Autodesk Fusion 360 part; units mm, degrees
(part 5 of 5)
equation "d1224 = DeckThick"
equation "d1226 = ( FootHeight ) + PanHeight - DeckThick"
equation "d1228 = ( BaseX + LeftRun + FaucetGap + RightRun - RightSideDepth ) + ( ( RightSideDepth ) - ( ( Wall + DeckClearance + RimBorder ) + ( ( RightSideDepth ) - 2 * ( Wall + DeckClearance + RimBorder ) ) ) )"
equation "d1229 = ( BaseY + Depth + ModuleGap ) + ( ( ( ( RightReach ) - ( 14 * SlotPitch + SlotWidth ) ) / 2 ) + ( 12 * SlotPitch ) )"
equation "d1230 = ( RightSideDepth ) - 2 * ( Wall + DeckClearance + RimBorder )"
equation "d1231 = SlotWidth"
equation "d1232 = DeckThick"
equation "d1234 = ( FootHeight ) + PanHeight - DeckThick"
equation "d1236 = ( BaseX + LeftRun + FaucetGap + RightRun - RightSideDepth ) + ( ( RightSideDepth ) - ( ( Wall + DeckClearance + RimBorder ) + ( ( RightSideDepth ) - 2 * ( Wall + DeckClearance + RimBorder ) ) ) )"
equation "d1237 = ( BaseY + Depth + ModuleGap ) + ( ( ( ( RightReach ) - ( 14 * SlotPitch + SlotWidth ) ) / 2 ) + ( 13 * SlotPitch ) )"
equation "d1238 = ( RightSideDepth ) - 2 * ( Wall + DeckClearance + RimBorder )"
equation "d1239 = SlotWidth"
equation "d1240 = DeckThick"
equation "d1242 = ( FootHeight ) + PanHeight - DeckThick"
equation "d1244 = ( BaseX + LeftRun + FaucetGap + RightRun - RightSideDepth ) + ( ( RightSideDepth ) - ( ( Wall + DeckClearance + RimBorder ) + ( ( RightSideDepth ) - 2 * ( Wall + DeckClearance + RimBorder ) ) ) )"
equation "d1245 = ( BaseY + Depth + ModuleGap ) + ( ( ( ( RightReach ) - ( 14 * SlotPitch + SlotWidth ) ) / 2 ) + ( 14 * SlotPitch ) )"
equation "d1246 = ( RightSideDepth ) - 2 * ( Wall + DeckClearance + RimBorder )"
equation "d1247 = SlotWidth"
equation "d1248 = DeckThick"
equation "d1250 = TouchChamfer"
equation "d1251 = FootHeight + PanHeight - DeckThick"
equation "d1253 = ( BaseX ) + ( ( Wall ) - DeckClearance )"
equation "d1254 = ( BaseY ) + ( 10 mm - DeckClearance )"
equation "d1255 = 2 mm + 2 * DeckClearance"
equation "d1256 = 5 mm + 2 * DeckClearance"
equation "d1257 = DeckThick"
equation "d1259 = FootHeight"
equation "d1261 = ( BaseX ) + ( Wall )"
equation "d1262 = ( BaseY ) + ( 10 mm )"
equation "d1265 = PanHeight"
equation "d1267 = FootHeight + PanHeight - DeckThick"
equation "d1269 = ( BaseX ) + ( ( ( TowerWidth ) - Wall - 2 mm ) - DeckClearance )"
equation "d1270 = ( BaseY ) + ( 10 mm - DeckClearance )"
equation "d1271 = 2 mm + 2 * DeckClearance"
equation "d1272 = 5 mm + 2 * DeckClearance"
equation "d1273 = DeckThick"
equation "d1275 = FootHeight"
equation "d1277 = ( BaseX ) + ( ( TowerWidth ) - Wall - 2 mm )"
equation "d1278 = ( BaseY ) + ( 10 mm )"
equation "d1281 = PanHeight"
equation "d1283 = FootHeight + PanHeight - DeckThick"
equation "d1285 = ( BaseX + TowerWidth + ModuleGap ) + ( ( Wall ) - DeckClearance )"
equation "d1286 = ( BaseY ) + ( 10 mm - DeckClearance )"
equation "d1287 = 2 mm + 2 * DeckClearance"
equation "d1288 = 5 mm + 2 * DeckClearance"
equation "d1289 = DeckThick"
equation "d1291 = FootHeight"
equation "d1293 = ( BaseX + TowerWidth + ModuleGap ) + ( Wall )"
equation "d1294 = ( BaseY ) + ( 10 mm )"
equation "d1297 = PanHeight"
equation "d1299 = FootHeight + PanHeight - DeckThick"
equation "d1301 = ( BaseX + TowerWidth + ModuleGap ) + ( ( ( LeftRun - TowerWidth - ModuleGap ) - Wall - 2 mm ) - DeckClearance )"
equation "d1302 = ( BaseY ) + ( 10 mm - DeckClearance )"
equation "d1303 = 2 mm + 2 * DeckClearance"
equation "d1304 = 5 mm + 2 * DeckClearance"
equation "d1305 = DeckThick"
equation "d1307 = FootHeight"
equation "d1309 = ( BaseX + TowerWidth + ModuleGap ) + ( ( LeftRun - TowerWidth - ModuleGap ) - Wall - 2 mm )"
equation "d1310 = ( BaseY ) + ( 10 mm )"
equation "d1313 = PanHeight"
equation "d1315 = FootHeight + PanHeight - DeckThick"
equation "d1317 = ( BaseX + LeftRun + FaucetGap ) + ( ( Wall ) - DeckClearance )"
equation "d1318 = ( BaseY ) + ( 10 mm - DeckClearance )"
equation "d1319 = 2 mm + 2 * DeckClearance"
equation "d1320 = 5 mm + 2 * DeckClearance"
equation "d1321 = DeckThick"
equation "d1323 = FootHeight"
equation "d1325 = ( BaseX + LeftRun + FaucetGap ) + ( Wall )"
equation "d1326 = ( BaseY ) + ( 10 mm )"
equation "d1329 = PanHeight"
equation "d1331 = FootHeight + PanHeight - DeckThick"
equation "d1333 = ( BaseX + LeftRun + FaucetGap ) + ( ( ( ( RightRun - ModuleGap ) / 2 ) - Wall - 2 mm ) - DeckClearance )"
equation "d1334 = ( BaseY ) + ( 10 mm - DeckClearance )"
equation "d1335 = 2 mm + 2 * DeckClearance"
equation "d1336 = 5 mm + 2 * DeckClearance"
equation "d1337 = DeckThick"
equation "d1339 = FootHeight"
equation "d1341 = ( BaseX + LeftRun + FaucetGap ) + ( ( ( RightRun - ModuleGap ) / 2 ) - Wall - 2 mm )"
equation "d1342 = ( BaseY ) + ( 10 mm )"
equation "d1345 = PanHeight"
equation "d1347 = FootHeight + PanHeight - DeckThick"
equation "d1349 = ( BaseX + LeftRun + FaucetGap + ( RightRun + ModuleGap ) / 2 ) + ( ( Wall ) - DeckClearance )"
equation "d1350 = ( BaseY ) + ( 10 mm - DeckClearance )"
equation "d1351 = 2 mm + 2 * DeckClearance"
equation "d1352 = 5 mm + 2 * DeckClearance"
equation "d1353 = DeckThick"
equation "d1355 = FootHeight"
equation "d1357 = ( BaseX + LeftRun + FaucetGap + ( RightRun + ModuleGap ) / 2 ) + ( Wall )"
equation "d1358 = ( BaseY ) + ( 10 mm )"
equation "d1361 = PanHeight"
equation "d1363 = FootHeight + PanHeight - DeckThick"
equation "d1365 = ( BaseX + LeftRun + FaucetGap + ( RightRun + ModuleGap ) / 2 ) + ( ( ( ( RightRun - ModuleGap ) / 2 ) - Wall - 2 mm ) - DeckClearance )"
equation "d1366 = ( BaseY ) + ( 10 mm - DeckClearance )"
equation "d1367 = 2 mm + 2 * DeckClearance"
equation "d1368 = 5 mm + 2 * DeckClearance"
equation "d1369 = DeckThick"
equation "d1371 = FootHeight"
equation "d1373 = ( BaseX + LeftRun + FaucetGap + ( RightRun + ModuleGap ) / 2 ) + ( ( ( RightRun - ModuleGap ) / 2 ) - Wall - 2 mm )"
equation "d1374 = ( BaseY ) + ( 10 mm )"
equation "d1377 = PanHeight"
equation "d1379 = FootHeight + PanHeight - DeckThick"
equation "d1381 = ( BaseX ) + ( 10 mm - DeckClearance )"
equation "d1382 = ( BaseY + Depth + ModuleGap ) + ( ( LeftReach ) - ( ( ( Wall ) - DeckClearance ) + ( 2 mm + 2 * DeckClearance ) ) )"
equation "d1383 = 5 mm + 2 * DeckClearance"
equation "d1384 = 2 mm + 2 * DeckClearance"
equation "d1385 = DeckThick"
equation "d1387 = FootHeight"
equation "d1389 = ( BaseX ) + ( 10 mm )"
equation "d1390 = ( BaseY + Depth + ModuleGap ) + ( ( LeftReach ) - ( ( Wall ) + ( 2 mm ) ) )"
equation "d1393 = PanHeight"
equation "d1395 = FootHeight + PanHeight - DeckThick"
equation "d1397 = ( BaseX ) + ( 10 mm - DeckClearance )"
equation "d1398 = ( BaseY + Depth + ModuleGap ) + ( ( LeftReach ) - ( ( ( ( LeftReach ) - Wall - 2 mm ) - DeckClearance ) + ( 2 mm + 2 * DeckClearance ) ) )"
equation "d1399 = 5 mm + 2 * DeckClearance"
equation "d1400 = 2 mm + 2 * DeckClearance"
equation "d1401 = DeckThick"
equation "d1403 = FootHeight"
equation "d1405 = ( BaseX ) + ( 10 mm )"
equation "d1406 = ( BaseY + Depth + ModuleGap ) + ( ( LeftReach ) - ( ( ( LeftReach ) - Wall - 2 mm ) + ( 2 mm ) ) )"
equation "d1409 = PanHeight"
equation "d1411 = FootHeight + PanHeight - DeckThick"
equation "d1413 = ( BaseX + LeftRun + FaucetGap + RightRun - RightSideDepth ) + ( ( RightSideDepth ) - ( ( 10 mm - DeckClearance ) + ( 5 mm + 2 * DeckClearance ) ) )"
equation "d1414 = ( BaseY + Depth + ModuleGap ) + ( ( Wall ) - DeckClearance )"
equation "d1415 = 5 mm + 2 * DeckClearance"
equation "d1416 = 2 mm + 2 * DeckClearance"
equation "d1417 = DeckThick"
equation "d1419 = FootHeight"
equation "d1421 = ( BaseX + LeftRun + FaucetGap + RightRun - RightSideDepth ) + ( ( RightSideDepth ) - ( ( 10 mm ) + ( 5 mm ) ) )"
equation "d1422 = ( BaseY + Depth + ModuleGap ) + ( Wall )"
equation "d1425 = PanHeight"
equation "d1427 = FootHeight + PanHeight - DeckThick"
equation "d1429 = ( BaseX + LeftRun + FaucetGap + RightRun - RightSideDepth ) + ( ( RightSideDepth ) - ( ( 10 mm - DeckClearance ) + ( 5 mm + 2 * DeckClearance ) ) )"
equation "d1430 = ( BaseY + Depth + ModuleGap ) + ( ( ( RightReach ) - Wall - 2 mm ) - DeckClearance )"
equation "d1431 = 5 mm + 2 * DeckClearance"
equation "d1432 = 2 mm + 2 * DeckClearance"
equation "d1433 = DeckThick"
equation "d1435 = FootHeight"
equation "d1437 = ( BaseX + LeftRun + FaucetGap + RightRun - RightSideDepth ) + ( ( RightSideDepth ) - ( ( 10 mm ) + ( 5 mm ) ) )"
equation "d1438 = ( BaseY + Depth + ModuleGap ) + ( ( RightReach ) - Wall - 2 mm )"
equation "d1441 = PanHeight"
named bodies: "R1_Integrated", "R1_RemovableGrate", "L1_Integrated", "L1_RemovableGrate", "L2_Integrated", "L2_RemovableGrate", "R2_Integrated", "R2_RemovableGrate", "LS_Integrated", "LS_RemovableGrate", "RS_Integrated", "RS_RemovableGrate"
